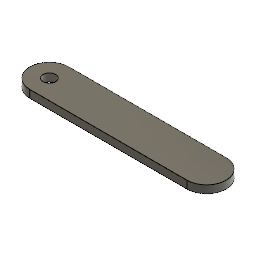
arm_2 v3 (Autodesk Fusion 360 design; units mm, degrees)
Autodesk Fusion 360 part; units mm, degrees
sketch "Sketch1" plane through (0, 0, 0) normal (0, 1, 0) x (1, 0, 0)
  circle A0 centre (-100, 0) radius 12.5
  circle A1 centre (-100, 0) radius 4
  circle A2 centre (0, 0) radius 12.5
  line L0 (0, 0) -> (0, 12.5)
  line L1 (0, 12.5) -> (-100, 12.5)
  line L2 (0, 0) -> (0, -2)
  line L3 (0, -2) -> (0, -12.5)
  line L4 (0, -12.5) -> (-100, -12.5)
  dimension "d2" = 25
  dimension "d16" = 8
  dimension "d19" = 25
  measures "d2" diameter of A0
  measures "d16" diameter of A1
  measures "d19" diameter of A2
extrude "Extrude2" add sketch "Sketch1" along normal blind 5 contours A0 | A1 makes body 1
extrude "Extrude1" add sketch "Sketch1" along normal blind 5 separate body contours A0 | A1 makes body 2
extrude "Extrude3" cut sketch "Sketch1" along normal blind 6 contours A1 bodies 1 2
extrude "Extrude4" add sketch "Sketch1" along normal blind 5 contours A0 A2 L1 L4 | A2 L0 L2 L3 | A2 L0 L2 L3 bodies 1 2
